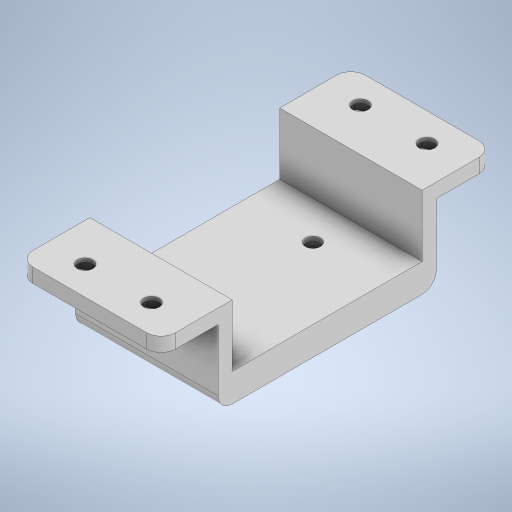
# Autodesk Inventor part: креп_камеры_ros
Saved by Autodesk Inventor 2024 (Build 280153000, 153)
## iProperties
Created: 2026-03-05
Part Number: креп_камеры_ros
Material: Типовые
Document SubType Name: Modeling
Designer: ejenie
Density: 1 g/cm^3
Appearance: По умолчанию
Author: ejenie
Autodesk Inventor part; units mm, degrees
ref_plane "YZ Plane" through (0, 0, 0) normal (1, 0, 0) x (0, 1, 0)
ref_plane "XZ Plane" through (0, 0, 0) normal (0, 1, 0) x (-1, 0, 0)
ref_plane "XY Plane" through (0, 0, 0) normal (0, 0, 1) x (1, 0, 0)
sketch "Эскиз1" plane through (0, 0, 0) normal (0, 1, 0) x (-1, 0, 0)
  line L0 (-15, 20) -> (15, 20)
  line L1 (15, 20) -> (15, -20)
  line L2 (15, -20) -> (-15, -20)
  line L3 (-15, -20) -> (-15, 20)
  line L4 (-15, 20) -> (15, -20) construction
  line L5 (15, 20) -> (-15, -20) construction
  point P0 (0, 0)
  dimension "d0" = 40
  dimension "d1" = 30
  constraints: 12 end point, 2 midpoint, 2 parallel, 1 horizontal, 1 perpendicular
  measures "d0" distance of L0.end L1.end
  measures "d1" distance of L1.end L2.end
extrude "Выдавливание1" add sketch "Эскиз1" along normal blind 6
sketch "Эскиз2" plane through (-15, 0, 20) normal (0, 0, 1) x (1, 0, 0)
  line L0 (30, 0) -> (0, 0) projected
  line L1 (0, 0) -> (30, 0)
  line L2 (30, 0) -> (30, 19)
  line L3 (30, 19) -> (0, 19)
  line L4 (0, 19) -> (0, 0)
  line L5 (0, 6) -> (30, 6) projected
  point P0 (15, 0)
  dimension "d4" = 13
  constraints: 8 end point, 2 parallel, 1 horizontal, 1 perpendicular
  measures "d4" distance between parallel lines of L5 L3
extrude "Выдавливание2" add sketch "Эскиз2" along normal blind 3
sketch "Эскиз4" plane through (-15, 19, 20) normal (0, 1, 0) x (1, 0, 0)
  line L0 (0, 40) -> (0, 0) projected
  line L1 (0, 0) -> (30, 0)
  line L2 (30, 0) -> (30, -15)
  line L3 (30, -15) -> (0, -15)
  line L4 (0, -15) -> (0, 0)
  point P0 (15, 20)
  point P1 (30, 0)
  dimension "d7" = 15
  constraints: 8 end point, 2 parallel, 1 horizontal, 1 perpendicular, 1 point on line
  measures "d7" distance between parallel lines of L1 L3
extrude "Выдавливание3" add sketch "Эскиз4" against normal blind 3
fillet "Сопряжение1" radius 3 3 edges at (15, 17.5, 35) (-15, 17.5, 35) (0, 0, 23)
sketch "Эскиз5" plane through (-15, 19, 20) normal (0, 1, 0) x (1, 0, 0)
  circle A0 centre (8, -9) radius 1.65
  circle A1 centre (22, -9) radius 1.65
  line L0 (0, 0) -> (0, -12) projected
  line L1 (30, -3) -> (30, -12) projected
  line L2 (30, 0) -> (0, 0) projected
  point P0 (15, 20)
  dimension "d11" = 3.3
  dimension "d12" = 3.3
  dimension "d13" = 8
  dimension "d14" = 8
  dimension "d15" = 9
  dimension "d16" = 9
  constraints: 2 centre point
  measures "d11" diameter of A0
  measures "d12" diameter of A1
  measures "d13" distance from line of L1 A1.centre
  measures "d14" distance from line of L0 A0.centre
  measures "d15" distance from line of A0.centre L2
  measures "d16" distance from line of L2 A1.centre
extrude "Выдавливание4" cut sketch "Эскиз5" against normal blind 3
sketch "Эскиз6" plane through (-15, 16, 20) normal (0, -1, 0) x (1, 0, 0)
  circle A0 centre (22, 9) radius 1.65 construction
  circle A1 centre (8, 9) radius 1.65 construction
  line L0 (24.75, 7.4123) -> (22, 5.8246)
  line L1 (22, 5.8246) -> (19.25, 7.4123)
  line L2 (19.25, 7.4123) -> (19.25, 10.5877)
  line L3 (19.25, 10.5877) -> (22, 12.1754)
  line L4 (22, 12.1754) -> (24.75, 10.5877)
  line L5 (24.75, 10.5877) -> (24.75, 7.4123)
  line L6 (10.75, 7.4123) -> (8, 5.8246)
  line L7 (8, 5.8246) -> (5.25, 7.4123)
  line L8 (5.25, 7.4123) -> (5.25, 10.5877)
  line L9 (5.25, 10.5877) -> (8, 12.1754)
  line L10 (8, 12.1754) -> (10.75, 10.5877)
  line L11 (10.75, 10.5877) -> (10.75, 7.4123)
  line L12 (0, 12) -> (0, 3) projected
  line L13 (30, 3) -> (30, 12) projected
  point P0 (15, -20)
  point P1 (19.25, 9)
  dimension "d19" = 5.5
  dimension "d20" = 5.5
  constraints: 24 end point, 2 coincident, 2 parallel, 1 midpoint, 26 other
  measures "d19" distance from line of point (19.25, 9) L5
  measures "d20" distance between parallel lines of L8 L11
extrude "Выдавливание5" cut sketch "Эскиз6" against normal blind 2.2
mirror "Зеркальное отражение1" about plane through (0, 0, 0) normal (0, 0, 1) of "Выдавливание2", "Сопряжение1", "Выдавливание5", "Выдавливание4", "Выдавливание3"
sketch "Эскиз7" plane through (0, 0, 0) normal (0, -1, 0) x (1, 0, 0)
  circle A0 centre (0, 12) radius 2.1
  circle A1 centre (0, -12) radius 2.1
  point P0 (0, 0)
  dimension "d23" = 4.2
  dimension "d24" = 4.2
  dimension "d25" = 12
  dimension "d26" = 12
  constraints: 2 centre point
  measures "d23" diameter of A0
  measures "d24" diameter of A1
  measures "d25" distance of point (0, 0) A1.centre
  measures "d26" distance of point (0, 0) A0.centre
extrude "Выдавливание6" cut sketch "Эскиз7" against normal blind 5
sketch "Эскиз8" plane through (0, 5, 12) normal (0, -1, 0) x (1, 0, 0)
  circle A0 centre (0, 0) radius 1.6
  circle A1 centre (0, -24) radius 2.1 projected
  circle A2 centre (0, -24) radius 1.6
  point P0 (0, -12)
  dimension "d29" = 3.2
  dimension "d30" = 3.2
  constraints: 2 centre point, 1 coincident
  measures "d29" diameter of A0
  measures "d30" diameter of A2
extrude "Выдавливание7" cut sketch "Эскиз8" against normal blind 6 contours A0 | A2
